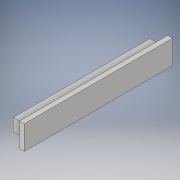
# Autodesk Inventor part: CardCover
Saved by Autodesk Inventor 2019 (Build 230136000, 136)
## iProperties
Created: 2021-04-26
Part Number: CardCover
Material: Všeobecné
Document SubType Name: Modeling
Designer: miko flosso
Density: 1 g/cm^3
Appearance: Výchozí
Author: miko flosso
Autodesk Inventor part; units mm, degrees
ref_plane "YZ Plane" through (0, 0, 0) normal (1, 0, 0) x (0, 1, 0)
ref_plane "XZ Plane" through (0, 0, 0) normal (0, 1, 0) x (-1, 0, 0)
ref_plane "XY Plane" through (0, 0, 0) normal (0, 0, 1) x (1, 0, 0)
sketch "Náčrt1" plane through (0, 0, 0) normal (1, 0, 0) x (0, 1, 0)
  line L0 (0, 0) -> (2.6, 0)
  line L1 (2.6, 0) -> (2.6, -28.6)
  line L2 (2.6, -28.6) -> (0, -28.6)
  line L3 (0, -28.6) -> (0, 0)
  dimension "d0" = 2.6
  dimension "d1" = 28.6
  constraints: 8 end point, 2 parallel, 1 horizontal, 1 perpendicular
  measures "d0" distance of L1.end L2.end
  measures "d1" distance of L0.end L1.end
extrude "Vysunutí1" add sketch "Náčrt1" along normal blind 2.5
sketch "Náčrt2" plane through (2.5, 0, 0) normal (1, 0, 0) x (0, 0, -1)
  line L0 (-1.2, -1.2) -> (29.8, -1.2)
  line L1 (29.8, -1.2) -> (29.8, 3.8)
  line L2 (29.8, 3.8) -> (-1.2, 3.8)
  line L3 (-1.2, 3.8) -> (-1.2, -1.2)
  line L4 (-1.2, -1.2) -> (29.8, 3.8) construction
  line L5 (29.8, -1.2) -> (-1.2, 3.8) construction
  line L6 (28.6, 2.6) -> (0, 2.6) projected
  point P0 (0, 0)
  point P1 (14.3, 1.3)
  dimension "d4" = 31
  dimension "d5" = 5
  dimension "d6" = 1.2
  constraints: 12 end point, 2 midpoint, 2 parallel, 1 horizontal, 1 perpendicular
  measures "d4" distance of L2.end L1.end
  measures "d5" distance of L1.end L0.end
  measures "d6" distance between parallel lines of L6 L2
extrude "Vysunutí2" add sketch "Náčrt2" along normal blind 1
